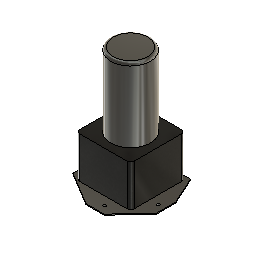
Motor c Suporte v3 (Autodesk Fusion 360 design; units mm, degrees)
Autodesk Fusion 360 part; units mm, degrees
sketch "Esboço1" plane through (0, 0, 0) normal (0, 0, 1) x (1, 0, 0)
  line L0 (30.5, -30.5) -> (-30.5, -30.5)
  line L1 (-30.5, -30.5) -> (-30.5, 30.5)
  line L2 (-30.5, 30.5) -> (30.5, 30.5)
  line L3 (30.5, 30.5) -> (30.5, -30.5)
  line L4 (30.5, -30.5) -> (-30.5, 30.5) construction
  line L5 (-30.5, -30.5) -> (30.5, 30.5) construction
  circle A0 centre (0, 0) radius 22.075
  dimension "d1" = 61
  dimension "d2" = 44.15
  constraint horizontal L0
  constraint perpendicular L0 L1
  constraint parallel L0 L2
  constraint parallel L1 L3
  constraint coincident L4 A0.centre
  constraint coincident L5 A0.centre
  constraint coincident A0.centre origin
  constraint equal L1 L2
  measures "d1" distance of L0.end L1.end
  measures "d2" diameter of A0
extrude "Extrusão1" add sketch "Esboço1" along normal blind 46.1
extrude "Extrusão2" add sketch "Esboço1" along normal blind 128.3 contours A0
fillet "Arredondamento1" radius 4 4 edges at (30.5, -30.5, 23.05) (30.5, 30.5, 23.05) (-30.5, 30.5, 23.05) (-30.5, -30.5, 23.05)
fillet "Arredondamento2" radius 3 1 edges at (-20.5811, -7.9827, 128.3)
sketch "Esboço3" plane through (0, 0, 0) normal (0, 0, 1) x (1, 0, 0)
sketch "Esboço4" plane through (0, 0, 0) normal (0, 0, 1) x (1, 0, 0)
  line L0 (-38.1983, -26.2505) -> (-1.3738, -48.4531)
  line L1 (-1.3738, -48.4531) -> (18.8762, -48.4531)
  line L2 (18.8762, -48.4531) -> (47.1993, -18.8085)
  line L3 (47.1993, -18.8085) -> (47.1993, 3.1915)
  line L4 (47.1993, 3.1915) -> (33.3001, 33.6725)
  line L5 (33.3001, 33.6725) -> (-38.1999, 33.6725)
  line L6 (-38.1999, 33.6725) -> (-38.1983, -26.2505)
  circle A0 centre (-25, -10) radius 1.5
  circle A1 centre (11, -40) radius 1.5
  circle A2 centre (40, -9) radius 1.5
  circle A3 centre (11, -40) radius 3
  circle A4 centre (40, -9) radius 3
  circle A5 centre (-25, -10) radius 3
  dimension "d25" = 3
  dimension "d26" = 3
  dimension "d27" = 3
  dimension "d28" = 20.25
  dimension "d29" = 43
  dimension "d30" = 71.5
  dimension "d31" = 33.5004
  dimension "d32" = 22
  dimension "d33" = 41
  dimension "d38" = 6
  dimension "d39" = 6
  dimension "d40" = 6
  constraint horizontal L1
  constraint perpendicular L1 L3
  constraint perpendicular L3 L5
  constraint concentric A1 A3
  constraint concentric A2 A4
  constraint concentric A0 A5
  measures "d25" diameter of A0
  measures "d26" diameter of A1
  measures "d27" diameter of A2
  measures "d28" distance of L0.end L1.end
  measures "d29" distance of L0.start L0.end
  measures "d30" distance of L4.end L5.end
  measures "d31" distance of L3.end L4.end
  measures "d32" distance of L2.end L3.end
  measures "d33" distance of L1.end L2.end
  measures "d38" diameter of A3
  measures "d39" diameter of A4
  measures "d40" diameter of A5
extrude "Extrusão5" add sketch "Esboço4" against normal blind 1 contours L0 L1 L2 L3 L4 L5 L6 | A3 | A4 | A5
extrude "Extrusão6" add sketch "Esboço4" against normal blind 4 contours A3 | A4 | A5
sketch "Esboço5" plane through (0, 0, -1) normal (0, 0, -1) x (1, 0, 0)
  circle A0 centre (40, 9) radius 3
  circle A1 centre (-25, 10) radius 3
  circle A2 centre (11, 40) radius 3
  line L0 (-38.1983, 26.2505) -> (-38.1999, -33.6725)
  line L1 (-38.1999, -33.6725) -> (33.3001, -33.6725)
  line L2 (33.3001, -33.6725) -> (47.1993, -3.1915)
  line L3 (47.1993, -3.1915) -> (47.1993, 18.8085)
  line L4 (47.1993, 18.8085) -> (18.8762, 48.4531)
  line L5 (18.8762, 48.4531) -> (-1.3738, 48.4531)
  line L6 (-1.3738, 48.4531) -> (-38.1983, 26.2505)
  line L7 (-1.3738, 48.4531) -> (-1.3738, 10) construction
  line L8 (-1.3738, 10) -> (-25, 10) construction
  line L9 (-5.3738, 10) -> (-4.3738, 10) construction
  line L10 (-4.3738, 10) -> (-4.3738, 7.3542)
  line L11 (-4.3738, 10) -> (-4.3738, 12.6458)
  arc A3 (-4.3738, 7.3542) -> (-4.3738, 12.6458) centre (-1.3738, 10) ccw
  dimension "d47" = 8
  dimension "d48" = 1
  constraint coincident L5.end L6.start
  constraint perpendicular L5 L7
  constraint coincident A1.centre L8.end
  constraint perpendicular L7 L8
  constraint coincident L7.end L8.start
  constraint coincident L8 L9.start
  constraint perpendicular L3 L9
  constraint perpendicular L8 L10
  constraint perpendicular L8 L11
  measures "d47" diameter of A3
  measures "d48" distance of L9.start L9.end
extrude "Extrusão8" add sketch "Esboço5" along normal blind 16 contours L10 L11 A3
equation "d5 = 46.1 mm + 82.2 mm"
